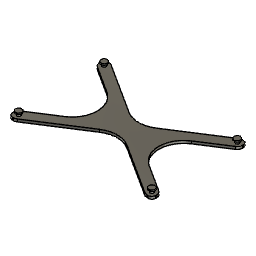
housing_holder (Autodesk Fusion 360 design; units mm, degrees)
Autodesk Fusion 360 part; units mm, degrees
sketch "Skizze1" plane through (0, 0, 0) normal (0, 0, 1) x (1, 0, 0)
  line L0 (0, 0) -> (57, 0)
  line L1 (57, 0) -> (57, 38)
  line L2 (57, 38) -> (0, 38)
  line L3 (0, 38) -> (0, 0)
  dimension "d1" = 57
  dimension "d2" = 38
  constraint horizontal L0
  constraint vertical L1
  constraint horizontal L2
  constraint vertical L3
  constraint coincident L0.start L3.end
  measures "d1" distance of L0.start L0.end
  measures "d2" distance of L0.start L2.end
extrude "Extrusion1" add sketch "Skizze1" along normal blind 1
sketch "Skizze2" plane through (0, 0, 1) normal (0, 0, 1) x (-1, 0, 0)
  line L0 (0, -38) -> (0, 0)
  line L1 (0, 0) -> (-57, 0)
  line L2 (-57, 0) -> (-57, -38)
  line L3 (-57, -38) -> (0, -38)
  circle A0 centre (-2, -36) radius 0.75
  circle A1 centre (-55, -36) radius 0.75
  circle A2 centre (-2, -2) radius 0.75
  circle A3 centre (-55, -2) radius 0.75
  line L4 (-2, -36) -> (-55, -36) construction
  line L5 (-55, -36) -> (-55, -2) construction
  line L6 (-55, -2) -> (-2, -2) construction
  line L7 (-2, -2) -> (-2, -36) construction
  line L8 (-28.5, -38) -> (-28.5, 0) construction
  line L9 (0, -19) -> (-57, -19) construction
  dimension "d5" = 1.5
  dimension "d6" = 1.5
  dimension "d7" = 1.5
  dimension "d8" = 1.5
  dimension "d9" = 53
  dimension "d10" = 53
  dimension "d11" = 26.5
  dimension "d12" = 17
  dimension "d13" = 34
  constraint coincident A0.centre L4.start
  constraint coincident A1.centre L4.end
  constraint perpendicular L2 L4
  constraint coincident A3.centre L5.end
  constraint coincident A2.centre L6.end
  constraint parallel L4 L6
  constraint vertical L7
  constraint midpoint L3 L8.start
  constraint midpoint L1 L8.end
  constraint midpoint L0 L9.start
  constraint midpoint L2 L9.end
  measures "d5" diameter of A0
  measures "d6" diameter of A1
  measures "d7" diameter of A2
  measures "d8" diameter of A3
  measures "d9" distance of A2.centre A3.centre
  measures "d10" distance of A0.centre A1.centre
  measures "d11" distance of A0.centre L8
  measures "d12" distance of L4 L9
  measures "d13" distance of A1.centre A3.centre
extrude "Extrusion2" add sketch "Skizze2" along normal blind 1 contours A0 | A1 | A2 | A3
sketch "Skizze3" plane through (0, 0, 2) normal (0, 0, 1) x (-1, 0, 0)
  circle A0 centre (-2, -36) radius 0.75
  circle A1 centre (-2, -36) radius 1.25
  circle A2 centre (-55, -36) radius 1.25
  circle A3 centre (-2, -2) radius 1.25
  circle A4 centre (-55, -2) radius 1.25
  dimension "d16" = 2.5
  dimension "d17" = 2.5
  dimension "d18" = 2.5
  dimension "d19" = 2.5
  constraint concentric A0 A1
  measures "d16" diameter of A1
  measures "d17" diameter of A2
  measures "d18" diameter of A3
  measures "d19" diameter of A4
extrude "Extrusion3" add sketch "Skizze3" along normal blind 0.5 contours A0 | A1 | A2 | A3 | A4
sketch "Skizze4" plane through (0, 0, 1) normal (0, 0, 1) x (-1, 0, 0)
  circle A0 centre (-2, -2) radius 0.75
  circle A1 centre (-2, -36) radius 0.75
  circle A2 centre (-55, -2) radius 0.75
  circle A3 centre (-55, -36) radius 0.75
  line L0 (0, -38) -> (0, 0)
  line L1 (0, 0) -> (-57, 0)
  line L2 (-57, 0) -> (-57, -38)
  line L3 (-57, -38) -> (0, -38)
  circle A4 centre (-2, -36) radius 2
  circle A5 centre (-55, -36) radius 2
  circle A6 centre (-55, -2) radius 2
  circle A7 centre (-2, -2) radius 2
  line L4 (-53.6905, -37.5117) -> (-28.5, -21.3634)
  line L5 (-24.8068, -18.9959) -> (-0.9206, -3.6837)
  line L6 (-0.8123, -34.3908) -> (-24.8068, -18.9959)
  line L7 (-28.5019, -16.6251) -> (-53.92, -0.3167)
  line L8 (-56.0794, -34.3163) -> (-32.1954, -18.9945)
  line L9 (-28.5019, -16.6251) -> (-3.0799, -0.3166)
  line L10 (-3.3095, -37.5117) -> (-28.5, -21.3634)
  line L11 (-32.1954, -18.9945) -> (-56.0794, -3.6837)
  constraint concentric A1 A4
  constraint concentric A3 A5
  constraint tangent L2 A5
  constraint concentric A2 A6
  constraint tangent L2 A6
  constraint concentric A0 A7
  constraint tangent L1 A7
  constraint coincident A4 L6.start
  constraint coincident A6 L7.end
  constraint tangent A6 L6
  constraint coincident A4 L10.start
  constraint coincident A6 L11.end
  constraint tangent A6 L10
  constraint coincident A5 L4.start
  constraint coincident A7 L5.end
  constraint tangent A7 L4
  constraint coincident A5 L8.start
  constraint coincident A7 L9.end
  constraint tangent A7 L8
  constraint collinear L4 L5
  constraint coincident L7.start L8
  constraint collinear L6 L7
  constraint coincident L8.end L10
  constraint collinear L8 L9
  constraint collinear L10 L11
extrude "Extrusion4" cut sketch "Skizze4" against normal blind 4 contours L0 A4 A7 L5 L6 | L3 A4 A5 L4 L10 | L1 A6 A7 L7 L9 | L2 A5 A6 L8 L11
fillet "Abrundung1" radius 1.5 4 edges at (0, 0, 0.5) (57, 0, 0.5) (57, 38, 0.5) (0, 38, 0.5)
fillet "Abrundung2" radius 10 4 edges at (28.5019, 16.6251, 0.5) (24.8068, 18.9959, 0.5) (28.5, 21.3634, 0.5) (32.1954, 18.9945, 0.5)
